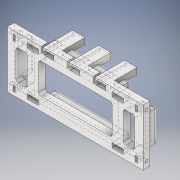
# Autodesk Inventor part: Batteryshelf
Saved by Autodesk Inventor 2019 (Build 230136000, 136)
## iProperties
Created: 2018-12-25
Part Number: Batteryshelf
Material: Generic
Document SubType Name: Modeling
Designer: Martin
Density: 1 g/cm^3
Appearance: Default
Author: Martin
Autodesk Inventor part; units mm, degrees
ref_plane "YZ Plane" through (0, 0, 0) normal (1, 0, 0) x (0, 1, 0)
ref_plane "XZ Plane" through (0, 0, 0) normal (0, 1, 0) x (-1, 0, 0)
ref_plane "XY Plane" through (0, 0, 0) normal (0, 0, 1) x (1, 0, 0)
sketch "Sketch1" plane through (0, 0, 0) normal (0, 0, 1) x (1, 0, 0)
  line L0 (-60, 25) -> (60, 25)
  line L1 (60, 25) -> (60, -25)
  line L2 (60, -25) -> (-60, -25)
  line L3 (-60, -25) -> (-60, 25)
  line L4 (-52.5, 17.5) -> (52.5, 17.5) construction
  line L5 (52.5, 17.5) -> (52.5, -17.5) construction
  line L6 (52.5, -17.5) -> (-52.5, -17.5) construction
  line L7 (-52.5, -17.5) -> (-52.5, 17.5) construction
  line L8 (-52.5, 17.5) -> (52.5, -17.5) construction
  line L9 (52.5, 17.5) -> (-52.5, -17.5) construction
  line L10 (-68.6467, 13.5) -> (97.7539, 13.5) construction
  line L11 (-76.5821, -13.5) -> (115.5782, -13.5) construction
  line L12 (-52.5, 13.5) -> (-56.5, 13.5)
  line L13 (-56.5, 13.5) -> (-56.5, -13.5)
  line L14 (-56.5, -13.5) -> (-52.5, -13.5)
  line L15 (-52.5, -13.5) -> (-52.5, 13.5)
  line L16 (52.5, 13.5) -> (56.5, 13.5)
  line L17 (56.5, 13.5) -> (56.5, -13.5)
  line L18 (56.5, -13.5) -> (52.5, -13.5)
  line L19 (52.5, -13.5) -> (52.5, 13.5)
  line L20 (-32.5, -39.2194) -> (-32.5, 40.0501) construction
  line L21 (32.5, -30.816) -> (32.5, 33.3794) construction
  line L22 (-32.5, -17.5) -> (32.5, -17.5)
  line L23 (32.5, -17.5) -> (32.5, -21.5)
  line L24 (32.5, -21.5) -> (-32.5, -21.5)
  line L25 (-32.5, -21.5) -> (-32.5, -17.5)
  line L26 (-32.5, 17.5) -> (32.5, 17.5)
  line L27 (32.5, 17.5) -> (32.5, 21.5)
  line L28 (32.5, 21.5) -> (-32.5, 21.5)
  line L29 (-32.5, 21.5) -> (-32.5, 17.5)
  line L30 (32.5, -21.5) -> (42.5, -21.5)
  line L31 (42.5, -21.5) -> (42.5, -17.5)
  line L32 (42.5, -17.5) -> (32.5, -17.5)
  line L33 (32.5, -17.5) -> (32.5, -21.5)
  line L34 (-32.5, -21.5) -> (-42.5, -21.5)
  line L35 (-42.5, -21.5) -> (-42.5, -17.5)
  line L36 (-42.5, -17.5) -> (-32.5, -17.5)
  line L37 (-32.5, -17.5) -> (-32.5, -21.5)
  line L38 (-32.5, 17.5) -> (-42.5, 17.5)
  line L39 (-42.5, 17.5) -> (-42.5, 21.5)
  line L40 (-42.5, 21.5) -> (-32.5, 21.5)
  line L41 (-32.5, 21.5) -> (-32.5, 17.5)
  line L42 (32.5, 17.5) -> (42.5, 17.5)
  line L43 (42.5, 17.5) -> (42.5, 21.5)
  line L44 (42.5, 21.5) -> (32.5, 21.5)
  line L45 (32.5, 21.5) -> (32.5, 17.5)
  point P0 (0, 0)
  dimension "d0" = 120
  dimension "d1" = 50
  dimension "d2" = 60
  dimension "d3" = 25
  dimension "d6" = 105
  dimension "d7" = 35
  dimension "d8" = 4
  dimension "d9" = 4
  dimension "d10" = 4
  dimension "d11" = 4
  dimension "d12" = 27
  dimension "d16" = 20
  dimension "d17" = 20
  dimension "d18" = 4
  dimension "d19" = 4
  dimension "d22" = 10
  dimension "d23" = 4
  dimension "d24" = 10
  dimension "d25" = 10
  dimension "d26" = 10
  constraints: 92 end point, 20 parallel, 12 horizontal, 12 point on line, 10 perpendicular, 2 midpoint, 2 vertical
  measures "d0" distance of L1.end L2.end
  measures "d1" distance of L0.end L1.end
  measures "d2" distance from line of point (0, 0) L3
  measures "d3" distance from line of point (0, 0) L0
  measures "d6" distance of L5.end L6.end
  measures "d7" distance of L4.end L5.end
  measures "d8" distance between parallel lines of L10 L4
  measures "d9" distance between parallel lines of L6 L11
  measures "d10" distance of L14.end L13.end
  measures "d11" distance of L17.end L18.end
  measures "d12" distance of L16.end L17.end
  measures "d16" distance between parallel lines of L7 L20
  measures "d17" distance between parallel lines of L5 L21
  measures "d18" distance of L22.end L23.end
  measures "d19" distance of L27.end L26.end
  measures "d22" distance of L32.end L31.end
  measures "d23" distance of L31.end L30.end
  measures "d24" distance of L35.end L36.end
  measures "d25" distance of L39.end L40.end
  measures "d26" distance of L44.end L43.end
extrude "Extrusion1" add sketch "Sketch1" along normal blind 6 contours L0 L1 L2 L3 | L15 L14 L13 L12 | L16 L17 L18 L19 | L22 L23 L24 L25 | L25 L34 L35 L36 | L32 L31 L30 L23 | L29 L28 L27 L26 | L38 L39 L40 L29 | L27 L44 L43 L42
extrude "Extrusion3" add sketch "Sketch1" against normal blind 10 contours L15 L14 L13 L12 | L16 L17 L18 L19 | L22 L23 L24 L25 | L29 L28 L27 L26
extrude "Extrusion4" cut sketch "Sketch1" along normal blind 10 contours L25 L34 L35 L36 | L32 L31 L30 L23 | L38 L39 L40 L29 | L27 L44 L43 L42
fillet "Fillet1" radius 2 16 edges at (0, -17.5, -10) (32.5, -19.5, -10) (0, -21.5, -10) (-32.5, -19.5, -10) (0, 17.5, -10) (-32.5, 19.5, -10) (0, 21.5, -10) (32.5, 19.5, -10) (-54.5, 13.5, -10) (-52.5, 0, -10) (-54.5, -13.5, -10) (-56.5, 0, -10) (54.5, 13.5, -10) (56.5, 0, -10) (54.5, -13.5, -10) (52.5, 0, -10)
sketch "Sketch2" plane through (60, -25, 0) normal (1, 0, 0) x (0, 0, -1)
  line L0 (0, 46.5) -> (-6, 46.5) construction
  line L1 (0, 42.5) -> (-6, 42.5) construction
  line L2 (0, 46.5) -> (-6, 46.5) construction
  line L3 (-6, 46.5) -> (-6, 42.5) construction
  line L4 (-6, 42.5) -> (0, 42.5) construction
  line L5 (0, 42.5) -> (0, 46.5) construction
  circle A0 centre (-3, 44.5) radius 1.25
  line L6 (0, 7.5) -> (8, 7.5) construction
  line L7 (0, 3.5) -> (-6, 3.5) construction
  line L8 (0, 7.5) -> (-6, 7.5) construction
  line L9 (-6, 7.5) -> (-6, 3.5) construction
  line L10 (-6, 3.5) -> (0, 3.5) construction
  line L11 (0, 3.5) -> (0, 7.5) construction
  circle A1 centre (-3, 5.5) radius 1.25
  point P0 (0, 25)
  point P1 (0, 11.5)
  point P2 (-6, 7.5)
  dimension "d30" = 2.5
  dimension "d32" = 2.5
  dimension "d65" = 3
  dimension "d66" = 3
  constraints: 16 end point, 4 parallel, 2 centre point, 2 horizontal, 2 perpendicular
  measures "d30" diameter of A0
  measures "d32" diameter of A1
  measures "d65" distance from line of A0.centre L5
  measures "d66" distance from line of A1.centre L11
extrude "Extrusion5" cut sketch "Sketch2" against normal blind 20
sketch "Sketch3" plane through (-60, -25, 0) normal (-1, 0, 0) x (0, 0, 1)
  line L0 (0, 3.5) -> (6, 3.5) construction
  line L1 (0, 7.5) -> (6, 7.5) construction
  line L2 (0, 3.5) -> (6, 3.5) construction
  line L3 (6, 3.5) -> (6, 7.5) construction
  line L4 (6, 7.5) -> (0, 7.5) construction
  line L5 (0, 7.5) -> (0, 3.5) construction
  line L6 (0, 42.5) -> (6, 42.5) construction
  line L7 (6, 46.5) -> (6, 42.5) construction
  line L8 (0, 42.5) -> (6, 42.5) construction
  line L9 (6, 42.5) -> (6, 46.5) construction
  line L10 (6, 46.5) -> (0, 46.5) construction
  line L11 (0, 46.5) -> (0, 42.5) construction
  circle A0 centre (3, 5.5) radius 1.25
  circle A1 centre (3, 44.5) radius 1.25
  point P0 (0, 25)
  dimension "d35" = 2.5
  dimension "d36" = 2.5
  dimension "d67" = 3
  dimension "d68" = 3
  constraints: 16 end point, 4 parallel, 2 centre point, 2 horizontal, 2 perpendicular
  measures "d35" diameter of A0
  measures "d36" diameter of A1
  measures "d67" distance from line of A0.centre L5
  measures "d68" distance from line of A1.centre L11
extrude "Extrusion6" cut sketch "Sketch3" against normal blind 20
sketch "Sketch4" plane through (0, 0, 0) normal (0, 0, -1) x (-1, 0, 0)
  line L0 (-55, 27.4058) -> (-55, -32.0223) construction
  line L1 (55, 25.9402) -> (55, -27.5524) construction
  line L2 (60, -25) -> (60, 25) projected
  line L3 (-60, 25) -> (-60, -25) projected
  line L4 (-60, 20.75) -> (-42.5, 20.75) construction
  line L5 (60, 25) -> (-60, 25) construction
  line L6 (-60, 19.5) -> (-42.9406, 19.5) construction
  line L7 (-55, 22) -> (-53.1, 22)
  line L8 (-53.1, 22) -> (-53.1, 17)
  line L9 (-53.1, 17) -> (-55, 17)
  line L10 (-55, 17) -> (-55, 22)
  line L11 (-55, -17) -> (-53.1, -17)
  line L12 (-53.1, -22) -> (-55, -22)
  line L13 (-55, -22) -> (-55, -17)
  line L14 (-53.1, -17) -> (-53.1, -22)
  line L15 (55, 22) -> (55, 17)
  line L16 (53.1, 22) -> (55, 22)
  line L17 (55, 17) -> (53.1, 17)
  line L18 (53.1, 17) -> (53.1, 22)
  line L19 (53.1, -17) -> (55, -17)
  line L20 (55, -17) -> (55, -22)
  line L21 (55, -22) -> (53.1, -22)
  line L22 (53.1, -22) -> (53.1, -17)
  line L23 (-60, -25) -> (-60, 25) projected
  point P0 (0, 0)
  point P1 (-60, 0)
  point P2 (60, 0)
  dimension "d39" = 5
  dimension "d40" = 5
  dimension "d45" = 1.25
  dimension "d46" = 1.9
  dimension "d47" = 5
  dimension "d48" = 2.5
  dimension "d51" = 39
  dimension "d58" = 108.1
  constraints: 38 end point, 3 horizontal, 3 parallel, 2 midpoint, 2 point on line, 2 vertical, 1 perpendicular, 24 other
  measures "d39" distance between parallel lines of L3 L0
  measures "d40" distance between parallel lines of L2 L1
  measures "d45" distance between parallel lines of L6 L4
  measures "d46" distance of L8.end L9.end
  measures "d47" distance of L7.end L8.end
  measures "d48" distance between parallel lines of L6 L7
  measures "d51" distance of L8.end L12.start
  measures "d58" distance of L7.end L15.start
extrude "Extrusion7" cut sketch "Sketch4" against normal blind 20
sketch "Sketch5" plane through (0, 0, 0) normal (0, 0, -1) x (-1, 0, 0)
  line L0 (-32.5, 17.5) -> (-32.5, -17.5) construction
  line L1 (32.5, 17.5) -> (32.5, -17.5) construction
  line L2 (60, -25) -> (60, 25) construction
  line L3 (-32.5, 17.5) -> (32.5, 17.5) construction
  line L4 (-52.7131, 13.4007) -> (52.2229, 13.4007) construction
  line L5 (-52.5, -13.5) -> (52.2229, -13.5) construction
  line L6 (-32.5, 13.4007) -> (32.5, 13.4007)
  line L7 (32.5, 13.4007) -> (32.5, -13.5)
  line L8 (32.5, -13.5) -> (-32.5, -13.5)
  line L9 (-32.5, -13.5) -> (-32.5, 13.4007)
  line L10 (-42.5, 17.5) -> (-42.5, -17.5) construction
  line L11 (42.5, 21.5) -> (42.5, 17.5) construction
  line L12 (42.5, 17.5) -> (42.5, -17.5) construction
  line L13 (52.5, -13.5) -> (52.5, 13.5) projected
  line L14 (42.5, 13.4007) -> (52.5, 13.4007)
  line L15 (52.5, 13.4007) -> (52.5, -13.5)
  line L16 (52.5, -13.5) -> (42.5, -13.5)
  line L17 (42.5, -13.5) -> (42.5, 13.4007)
  line L18 (-52.5, -13.5) -> (-52.5, 13.5) projected
  line L19 (-42.5, 13.4007) -> (-52.5, 13.4007)
  line L20 (-52.5, 13.4007) -> (-52.5, -13.5)
  line L21 (-52.5, -13.5) -> (-42.5, -13.5)
  line L22 (-42.5, -13.5) -> (-42.5, 13.4007)
  constraints: 36 end point, 8 point on line, 6 parallel, 5 horizontal, 4 vertical, 3 perpendicular
extrude "Extrusion9" cut sketch "Sketch5" against normal blind 20
fillet "Fillet4" radius 2 12 edges at (52.5, 13.4007, 3) (42.5, 13.4007, 3) (52.5, -13.5, 3) (42.5, -13.5, 3) (32.5, -13.5, 3) (32.5, 13.4007, 3) (-32.5, 13.4007, 3) (-32.5, -13.5, 3) (-42.5, 13.4007, 3) (-42.5, -13.5, 3) (-52.5, -13.5, 3) (-52.5, 13.4007, 3)
sketch "Sketch6" plane through (0, 0, 0) normal (0, 0, -1) x (-1, 0, 0)
  line L0 (30.5, 13.4007) -> (-30.5, 13.4007) projected
  line L1 (-4, 31.1432) -> (-4, 7.174) construction
  line L2 (4, 32.2222) -> (4, 4.5535) construction
  line L3 (-32.5, 17.5) -> (-30.5, 19.5) construction
  line L4 (-4, 23.5) -> (4, 23.5)
  line L5 (4, 23.5) -> (4, 19.5)
  line L6 (4, 19.5) -> (-4, 19.5)
  line L7 (-4, 19.5) -> (-4, 23.5)
  line L8 (32.5, 21.5) -> (-32.5, 21.5) construction
  line L9 (-4, 23.5) -> (4, 19.5)
  line L10 (4, 23.5) -> (-4, 19.5)
  line L11 (-5.5, 33.6047) -> (-5.5, 8.1256) construction
  line L12 (-60, 25) -> (60, 25) projected
  line L13 (-5.5, 25) -> (-4, 25)
  line L14 (-4, 25) -> (-4, 19.5)
  line L15 (-4, 19.5) -> (-5.5, 19.5)
  line L16 (-5.5, 19.5) -> (-5.5, 25)
  line L17 (-4, 25) -> (4, 25)
  line L18 (4, 25) -> (4, 23.5)
  line L19 (4, 23.5) -> (-4, 23.5)
  line L20 (-4, 23.5) -> (-4, 25)
  line L21 (4, 25) -> (5.5, 25)
  line L22 (5.5, 25) -> (5.5, 21.5)
  line L23 (5.5, 21.5) -> (4, 21.5)
  line L24 (4, 21.5) -> (4, 25)
  line L25 (4, 21.5) -> (5.5, 21.5)
  line L26 (5.5, 21.5) -> (5.5, 19.5)
  line L27 (4, 19.5) -> (4, 21.5)
  line L28 (-30.5, 19.5) -> (4, 19.5) construction
  line L29 (5.5, 19.5) -> (30.5, 19.5) construction
  line L30 (5.5, 34.5455) -> (5.5, 21.5) construction
  line L31 (5.5, 19.5) -> (5.5, 7.7728) construction
  line L32 (4, 21.5) -> (7, 21.5)
  line L33 (7, 21.5) -> (7, 20)
  line L34 (7, 20) -> (4, 20)
  line L35 (4, 20) -> (4, 21.5)
  line L36 (5.5, 21.5) -> (7, 21.5)
  line L37 (7, 21.5) -> (7, 25)
  line L38 (7, 25) -> (5.5, 25)
  line L39 (5.5, 25) -> (5.5, 21.5)
  line L40 (19, 23.5) -> (27, 23.5)
  line L41 (27, 19.5) -> (19, 19.5)
  line L42 (19, 19.5) -> (19, 23.5)
  line L43 (17.5, 25) -> (19, 25)
  line L44 (19, 23.5) -> (19, 19.5)
  line L45 (19, 19.5) -> (17.5, 19.5)
  line L46 (17.5, 19.5) -> (17.5, 25)
  line L47 (19, 25) -> (27, 25)
  line L48 (27, 23.5) -> (19, 23.5)
  line L49 (27, 25) -> (28.5, 25)
  line L50 (28.5, 25) -> (28.5, 21.5)
  line L51 (28.5, 21.5) -> (27, 21.5)
  line L52 (27, 21.5) -> (27, 23.5)
  line L53 (27, 21.5) -> (28.5, 21.5)
  line L54 (27, 19.5) -> (27, 20)
  line L55 (27, 21.5) -> (28.5, 21.5)
  line L56 (30, 21.5) -> (30, 20)
  line L57 (30, 20) -> (27, 20)
  line L58 (27, 20) -> (27, 21.5)
  line L59 (30, 21.5) -> (30, 25)
  line L60 (30, 25) -> (28.5, 25)
  line L61 (28.5, 25) -> (28.5, 21.5)
  line L62 (-27, 23.5) -> (-19, 23.5)
  line L63 (-19, 23.5) -> (-19, 19.5)
  line L64 (-19, 19.5) -> (-27, 19.5)
  line L65 (-27, 19.5) -> (-27, 23.5)
  line L66 (-28.5, 25) -> (-27, 25)
  line L67 (-27, 25) -> (-27, 19.5)
  line L68 (-27, 19.5) -> (-28.5, 19.5)
  line L69 (-28.5, 19.5) -> (-28.5, 25)
  line L70 (-27, 25) -> (-19, 25)
  line L71 (-19, 25) -> (-19, 23.5)
  line L72 (-19, 23.5) -> (-27, 23.5)
  line L73 (-27, 23.5) -> (-27, 25)
  line L74 (-19, 25) -> (-17.5, 25)
  line L75 (-17.5, 25) -> (-17.5, 21.5)
  line L76 (-17.5, 21.5) -> (-19, 21.5)
  line L77 (-19, 21.5) -> (-19, 25)
  line L78 (-19, 21.5) -> (-17.5, 21.5)
  line L79 (-19, 19.5) -> (-19, 21.5)
  line L80 (-19, 21.5) -> (-17.5, 21.5)
  line L81 (-16, 21.5) -> (-16, 20)
  line L82 (-16, 20) -> (-19, 20)
  line L83 (-19, 20) -> (-19, 21.5)
  line L84 (-16, 21.5) -> (-16, 25)
  line L85 (-16, 25) -> (-17.5, 25)
  line L86 (-17.5, 25) -> (-17.5, 21.5)
  line L87 (19, 23.5) -> (19, 19.5)
  line L88 (27, 23.5) -> (27, 21.5)
  line L89 (27, 20) -> (27, 19.5)
  line L90 (28.5, 25) -> (27, 25)
  line L91 (27, 23.5) -> (27, 21.5)
  line L92 (27, 21.5) -> (28.5, 21.5)
  line L93 (28.5, 21.5) -> (28.5, 25)
  line L94 (27, 23.5) -> (19, 23.5)
  line L95 (19, 23.5) -> (19, 19.5)
  line L96 (19, 19.5) -> (27, 19.5)
  line L97 (27, 19.5) -> (27, 23.5)
  line L98 (28.5, 21.5) -> (27, 21.5)
  line L99 (27, 21.5) -> (27, 20)
  line L100 (27, 20) -> (30, 20)
  line L101 (30, 20) -> (30, 21.5)
  line L102 (30, 25) -> (28.5, 25)
  line L103 (28.5, 25) -> (28.5, 21.5)
  line L104 (30, 21.5) -> (30, 25)
  line L105 (30, 25) -> (28.5, 25)
  line L106 (28.5, 21.5) -> (27, 21.5)
  line L107 (30, 25) -> (28.5, 25)
  line L108 (28.5, 25) -> (28.5, 20)
  line L109 (28.5, 20) -> (30, 20)
  line L110 (30, 20) -> (30, 25)
  line L111 (28.5, 20) -> (27, 20)
  line L112 (27, 20) -> (27, 21.5)
  line L113 (27, 21.5) -> (28.5, 21.5)
  line L114 (28.5, 21.5) -> (28.5, 20)
  line L115 (-17.5, 25) -> (-19, 25)
  line L116 (-19, 25) -> (-19, 21.5)
  line L117 (-19, 21.5) -> (-17.5, 21.5)
  line L118 (-17.5, 21.5) -> (-17.5, 25)
  line L119 (-19, 23.5) -> (-27, 23.5)
  line L120 (-27, 23.5) -> (-27, 25)
  line L121 (-27, 25) -> (-19, 25)
  line L122 (-19, 25) -> (-19, 23.5)
  line L123 (-27, 25) -> (-28.5, 25)
  line L124 (-28.5, 25) -> (-28.5, 19.5)
  line L125 (-28.5, 19.5) -> (-27, 19.5)
  line L126 (-27, 19.5) -> (-27, 25)
  line L127 (-19, 23.5) -> (-27, 23.5)
  line L128 (-27, 23.5) -> (-27, 19.5)
  line L129 (-27, 19.5) -> (-19, 19.5)
  line L130 (-19, 19.5) -> (-19, 23.5)
  line L131 (-16, 21.5) -> (-19, 21.5)
  line L132 (-19, 21.5) -> (-19, 20)
  line L133 (-19, 20) -> (-16, 20)
  line L134 (-16, 20) -> (-16, 21.5)
  line L135 (-16, 25) -> (-17.5, 25)
  line L136 (-17.5, 25) -> (-17.5, 21.5)
  line L137 (-17.5, 21.5) -> (-16, 21.5)
  line L138 (-16, 21.5) -> (-16, 25)
  line L139 (-19, 23.5) -> (-27, 23.5)
  line L140 (-27, 23.5) -> (-27, 19.5)
  line L141 (-27, 19.5) -> (-19, 19.5)
  line L142 (-19, 19.5) -> (-19, 23.5)
  point P0 (0, 0)
  point P1 (0, 21.5)
  dimension "d91" = 4
  dimension "d92" = 8
  dimension "d95" = 5.5
  dimension "d99" = 3
  dimension "d100" = 1.5
  dimension "d103" = 3
  dimension "d104" = 1.5
  dimension "d105" = 3
  dimension "d106" = 1.5
  dimension "d107" = 15
  dimension "d108" = 15
  constraints: 278 end point, 61 parallel, 34 horizontal, 30 perpendicular, 9 point on line, 5 vertical, 4 midpoint, 2 collinear
  measures "d91" distance from line of point (0, 0) L1
  measures "d92" distance between parallel lines of L2 L1
  measures "d95" distance from line of point (0, 0) L11
  measures "d99" distance of L33.end L34.end
  measures "d100" distance of L32.end L33.end
  measures "d103" distance of L57.end L57.start
  measures "d104" distance of L56.start L57.start
  measures "d105" distance of L82.start L82.end
  measures "d106" distance of L81.start L82.start
  measures "d107" distance between parallel lines of L42 L2
  measures "d108" distance between parallel lines of L63 L1
extrude "Extrusion10" cut sketch "Sketch6" along normal mid plane 40 contours L9 L10 L7 | L4 L10 L9 | L5 L9 L10 | L10 L9 L6
extrude "Extrusion11" add sketch "Sketch6" along normal blind 20 contours L14 L12 L18 L4 | L7 L15 L16 L12 L14 | L18 L12 L22 L23 L5
extrude "Extrusion12" cut sketch "Sketch6" along normal mid plane 30 contours L23 L26 L34 L5 | L32 L33 L34 L26 | L22 L12 L37 L32
extrude "Extrusion14" cut sketch "Sketch6" along normal mid plane 20 contours L42 L40 L52 L58 L54 L41
extrude "Extrusion15" add sketch "Sketch6" along normal blind 20 contours L12 L50 L51 L52 L40 L42 L45 L46
extrude "Extrusion16" cut sketch "Sketch6" along normal mid plane 20 contours L12 L59 L56 L57 L108 L50 | L108 L57 L58 L51
extrude "Extrusion17" add sketch "Sketch6" along normal blind 20 contours L75 L76 L63 L71 L12 | L71 L62 L67 L12 | L67 L65 L68 L69 L12
extrude "Extrusion18" cut sketch "Sketch6" along normal mid plane 20 contours L84 L131 L75 L12 | L81 L82 L63 L76 L131
sketch "Sketch7" plane through (0, 0, 6) normal (0, 0, 1) x (1, 0, 0)
  line L0 (19, 23.5) -> (19, 21.5) projected
  line L1 (27, 21.5) -> (27, 19.5) projected
  line L2 (19, 23.5) -> (27, 23.5)
  line L3 (27, 23.5) -> (27, 19.5)
  line L4 (27, 19.5) -> (19, 19.5)
  line L5 (19, 19.5) -> (19, 23.5)
  point P0 (0, 0)
  constraints: 8 end point, 2 parallel, 1 horizontal, 1 perpendicular
extrude "Extrusion19" cut sketch "Sketch7" against normal blind 20
equation "\"d2\" = 0.5 * d0"
equation "\"d3\" = 0.5 * d1"
equation "\"d66\" = d65"
equation "\"d68\" = d67"
equation "\"d48\" = 0.5 * d47"
equation "\"d92\" = 2 * d91"
equation "\"d108\" = d107"
equation "\"d96\" = d95"
body "Solid1"
